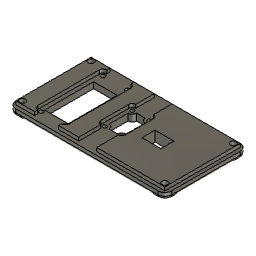
box+top (Autodesk Fusion 360 design; units mm, degrees)
Autodesk Fusion 360 part; units mm, degrees
note: some values were not read from the file. Set by a fixed rule: which face or edge a step refers to.
sketch "box dimensions" plane through (0, 0, 0) normal (0, 0, 1) x (1, 0, 0)
  line L0 (104.14, -1.27) -> (-6.35, -1.27)
  line L1 (-6.35, -1.27) -> (-6.35, 54.61)
  line L2 (-6.35, 54.61) -> (104.14, 54.61)
  line L3 (104.14, 54.61) -> (104.14, -1.27)
  line L4 (101.6, 57.15) -> (-3.81, 57.15)
  line L5 (-8.89, 52.07) -> (-8.89, 1.27)
  line L6 (-3.81, -3.81) -> (101.6, -3.81)
  arc A0 (106.68, 52.07) -> (101.6, 57.15) centre (101.6, 52.07) ccw
  line L7 (106.68, 1.27) -> (106.68, 52.07)
  arc A1 (-3.81, 57.15) -> (-8.89, 52.07) centre (-3.81, 52.07) ccw
  arc A2 (101.6, -3.81) -> (106.68, 1.27) centre (101.6, 1.27) ccw
  arc A3 (-8.89, 1.27) -> (-3.81, -3.81) centre (-3.81, 1.27) ccw
  circle A4 centre (-3.81, 52.07) radius 2.159
  circle A5 centre (-3.81, 1.27) radius 2.159
  circle A6 centre (101.6, 1.27) radius 2.159
  circle A7 centre (-3.81, 52.07) radius 2.159
  circle A8 centre (-3.81, 1.27) radius 2.159
  circle A9 centre (101.6, 52.07) radius 2.159
  line L8 (68.834, 6.35) -> (68.834, 4.9748)
  line L9 (-0.254, 53.594) -> (64.6598, 53.594)
  line L10 (71.12, 6.35) -> (68.834, 6.35)
  line L11 (-2.159, 2.921) -> (-2.159, 12.319)
  line L12 (104.14, 54.61) -> (-6.35, 54.61)
  line L13 (-2.159, 12.319) -> (-0.254, 12.319)
  line L14 (104.14, -1.27) -> (104.14, 54.61)
  line L15 (-0.254, -0.254) -> (-0.254, 2.921)
  line L16 (98.044, 0) -> (71.12, 0)
  line L17 (71.12, 53.34) -> (98.044, 53.34)
  line L18 (-6.35, 44.069) -> (-0.254, 44.069)
  line L19 (98.044, 53.34) -> (98.044, 0)
  line L20 (-6.35, -1.27) -> (104.14, -1.27)
  line L21 (-0.254, 30.861) -> (-6.35, 30.861)
  line L22 (66.294, -0.254) -> (-0.254, -0.254)
  line L23 (-0.254, 2.921) -> (-2.159, 2.921)
  line L24 (-0.254, 44.069) -> (-0.254, 53.594)
  line L25 (71.12, 0) -> (71.12, 6.35)
  line L26 (66.294, 2.4348) -> (66.294, -0.254)
  line L27 (71.12, 50.8704) -> (71.12, 53.34)
  line L28 (-0.254, 12.319) -> (-0.254, 30.861)
  line L29 (-6.35, 30.861) -> (-6.35, -1.27)
  line L30 (66.294, 50.8704) -> (71.12, 50.8704)
  line L31 (-6.35, 54.61) -> (-6.35, 44.069)
  line L32 (64.6598, 53.594) -> (66.294, 50.8704)
  line L33 (68.834, 4.9748) -> (66.294, 2.4348)
  circle A10 centre (101.6, 52.07) radius 2.159
  circle A11 centre (101.6, 1.27) radius 2.159
extrude "Extrude1" add sketch "box dimensions" along normal blind 2.54 contours L0 L1 L2 L3 L8 L9 L10 L11 L12 L13 L14 L15 L16 L17 L18 L19 L20 L21 L22 L23 L24 L25 L26 L27 L28 L29 L30 L31 L32 L33 | L1 L8 L9 L10 L11 L13 L15 L16 L17 L18 L19 L21 L22 L23 L24 L25 L26 L27 L28 L30 L32 L33 | L4 L5 L6 A0 L7 A1 A2 A3
extrude "Extrude2" add sketch "box dimensions" along normal blind 5.08 contours L0 L1 L2 L3 L8 L9 L10 L11 L12 L13 L14 L15 L16 L17 L18 L19 L20 L21 L22 L23 L24 L25 L26 L27 L28 L29 L30 L31 L32 L33 | L1 L8 L9 L10 L11 L13 L15 L16 L17 L18 L19 L21 L22 L23 L24 L25 L26 L27 L28 L30 L32 L33
move_face "OffsetFaces1" offset 2.54 1 faces at (65.8149, 18.5156, 0)
hole "Hole2" at (-3.81, 1.27, 0) at (-3.81, 52.07, 0) at (101.6, 52.07, 0) at (101.6, 1.27, 0) direction (0, 0, -1) diameter 8.763 depth 2.54 tip angle 180
fillet "Fillet1" radius 2.54 8 edges at (48.895, 57.15, -2.54) (-7.4021, 55.6621, -2.54) (-8.89, 26.67, -2.54) (-7.4021, -2.3221, -2.54) (48.895, -3.81, -2.54) (105.1921, -2.3221, -2.54) (106.68, 26.67, -2.54) (105.1921, 55.6621, -2.54) 1 faces at (32.5915, 34.4064, -2.54)
sketch "featherwing exact dimensions" plane through (0, 0, 5.08) normal (0, 0, 1) x (1, 0, 0)
  line L0 (25.4, 52.07) -> (7.62, 52.07)
  arc A0 (27.94, 49.53) -> (25.4, 52.07) centre (25.4, 49.53) ccw
  line L1 (27.94, 3.81) -> (27.94, 49.53)
  arc A1 (25.4, 1.27) -> (27.94, 3.81) centre (25.4, 3.81) ccw
  arc A2 (5.08, 3.81) -> (7.62, 1.27) centre (7.62, 3.81) ccw
  line L2 (5.08, 49.53) -> (5.08, 3.81)
  arc A3 (7.62, 52.07) -> (5.08, 49.53) centre (7.62, 49.53) ccw
  line L3 (7.62, 1.27) -> (25.4, 1.27)
  line L4 (25.019, 42.0878) -> (8.001, 42.0878)
  line L5 (25.019, 6.2992) -> (25.019, 42.0878)
  line L6 (8.001, 6.2992) -> (25.019, 6.2992)
  line L7 (8.001, 42.0878) -> (8.001, 6.2992)
  circle A4 centre (7.62, 49.53) radius 1.27
  circle A5 centre (25.4, 49.53) radius 1.27
  circle A6 centre (25.4, 3.81) radius 1.27
  circle A7 centre (7.62, 3.81) radius 1.27
  circle A8 centre (101.6, 1.27) radius 2.159
  circle A9 centre (101.6, 52.07) radius 2.159
  circle A10 centre (-3.81, 1.27) radius 2.159
  circle A11 centre (-3.81, 52.07) radius 2.159
  line L8 (-6.35, 54.61) -> (-6.35, -1.27)
  line L9 (-6.35, -1.27) -> (104.14, -1.27)
  line L10 (104.14, -1.27) -> (104.14, 54.61)
  line L11 (104.14, 54.61) -> (-6.35, 54.61)
  circle A12 centre (7.62, 49.53) radius 1.905
  circle A13 centre (25.4, 49.53) radius 1.905
  circle A14 centre (25.4, 3.81) radius 1.905
  circle A15 centre (7.62, 3.81) radius 1.905
  dimension "d75" = 3.81
  dimension "d76" = 3.81
  dimension "d77" = 3.81
  dimension "d78" = 3.81
  constraint concentric A3 A12
  constraint concentric A0 A13
  constraint concentric A6 A14
  constraint concentric A2 A15
  measures "d75" diameter of A12
  measures "d76" diameter of A13
  measures "d77" diameter of A14
  measures "d78" diameter of A15
extrude "Extrude3" cut sketch "featherwing exact dimensions" against normal blind 12.7 contours A4 | A5 | A6 | A7
extrude "Extrude4" cut sketch "featherwing exact dimensions" against normal blind 10.16 contours L4 L5 L6 L7
move_face "OffsetFaces2" offset -0.254 4 faces at (25.019, 18.2287, 2.54) (19.3463, 6.2992, 0) (8.001, 30.1583, 2.54) (13.6737, 42.0878, 0)
extrude "Extrude5" cut sketch "featherwing exact dimensions" against normal blind 5.08 contours L0 A0 L1 A1 A2 L2 A3 L3 | A12 | A13 | A14 | A15
move_face "OffsetFaces3" offset -0.254 4 faces at (27.94, 19.05, 3.3867) (13.5467, 52.07, 1.6933) (13.5467, 1.27, 3.3867) (5.08, 34.29, 3.3867)
move_face "OffsetFaces4" offset -0.254 4 faces at (26.6637, 3.6835, -0.8467) (26.6637, 49.4035, -0.8467) (8.8884, 49.5933, -0.8467) (8.8837, 3.6835, -0.8467)
sketch "aht20 exact dimensions" plane through (0, 0, 5.08) normal (0, 0, 1) x (1, 0, 0)
  line L0 (53.34, 40.64) -> (40.64, 40.64)
  line L1 (38.1, 38.1) -> (38.1, 17.78)
  line L2 (55.88, 17.78) -> (55.88, 38.1)
  arc A0 (38.1, 17.78) -> (40.64, 15.24) centre (40.64, 17.78) ccw
  arc A1 (55.88, 38.1) -> (53.34, 40.64) centre (53.34, 38.1) ccw
  arc A2 (53.34, 15.24) -> (55.88, 17.78) centre (53.34, 17.78) ccw
  arc A3 (40.64, 40.64) -> (38.1, 38.1) centre (40.64, 38.1) ccw
  line L3 (40.64, 15.24) -> (53.34, 15.24)
  circle A4 centre (40.64, 17.78) radius 1.27
  circle A5 centre (40.64, 38.1) radius 1.27
  circle A6 centre (53.34, 38.1) radius 1.27
  circle A7 centre (53.34, 17.78) radius 1.27
extrude "Extrude6" cut sketch "aht20 exact dimensions" against normal blind 2.54
extrude "Extrude7" cut 4 faces at (40.4853, 18.1741, 5.08) (40.8517, 37.7334, 5.08) (53.1853, 38.4392, 5.08) (53.1853, 18.1741, 5.08) along direction (0, 0, -1) blind 7.62
move_face "OffsetFaces5" offset -0.254 4 faces at (38.1, 31.3267, 4.2333) (44.8733, 15.24, 4.2333) (55.88, 24.5533, 3.3867) (49.1067, 40.64, 4.2333)
move_face "OffsetFaces6" offset -0.127 4 faces at (52.2563, 37.4378, -0.8467) (40.8605, 39.3507, 0.8467) (52.2563, 17.1178, -0.8467) (39.5563, 17.1178, -0.8467)
sketch "Sketch4" plane through (0, 0, 0) normal (0, 0, 1) x (-1, 0, 0)
  arc A0 (-4.826, -3.556) -> (-7.366, -1.016) centre (-7.366, -3.556) ccw
  line L0 (-7.366, -1.016) -> (-25.654, -1.016)
  arc A1 (-25.654, -1.016) -> (-28.194, -3.556) centre (-25.654, -3.556) ccw
  line L1 (-28.194, -3.556) -> (-28.194, -49.784)
  arc A2 (-28.194, -49.784) -> (-25.654, -52.324) centre (-25.654, -49.784) ccw
  line L2 (-25.654, -52.324) -> (-7.366, -52.324)
  arc A3 (-7.366, -52.324) -> (-4.826, -49.784) centre (-7.366, -49.784) ccw
  line L3 (-4.826, -49.784) -> (-4.826, -3.556)
  line L4 (-7.747, -42.3418) -> (-25.273, -42.3418)
  line L5 (-25.273, -42.3418) -> (-25.273, -6.0452)
  line L6 (-25.273, -6.0452) -> (-7.747, -6.0452)
  line L7 (-7.747, -6.0452) -> (-7.747, -42.3418)
  circle A4 centre (-7.62, -3.81) radius 1.524
  circle A5 centre (-25.4, -49.53) radius 1.524
  circle A6 centre (-7.62, -49.53) radius 1.524
  circle A7 centre (-25.4, -3.81) radius 1.524
  point P0 (-53.34, -38.1)
  point P1 (-40.64, -38.1)
  point P2 (-40.64, -17.78)
  point P3 (-53.34, -17.78)
hole "Hole3" at (53.34, 17.78, 0) at (53.34, 38.1, 0) at (40.64, 17.78, 0) at (40.64, 38.1, 0) direction (0, 0, -1) diameter 7.62 depth 2.54 tip angle 180
sketch "Sketch5" plane through (0, 0, -2.54) normal (0, 0, -1) x (1, 0, 0)
  circle A0 centre (40.64, -17.78) radius 3.81
  circle A1 centre (53.34, -17.78) radius 3.81
  circle A2 centre (53.34, -38.1) radius 3.81
  circle A3 centre (40.64, -38.1) radius 3.81
  line L0 (7.747, -6.0452) -> (25.273, -6.0452)
  line L1 (25.273, -6.0452) -> (25.273, -42.3418)
  line L2 (25.273, -42.3418) -> (7.747, -42.3418)
  line L3 (7.747, -42.3418) -> (7.747, -6.0452)
  circle A4 centre (25.4, -3.81) radius 1.524
  circle A5 centre (25.4, -49.53) radius 1.524
  circle A6 centre (7.62, -3.81) radius 1.524
  circle A7 centre (7.62, -49.53) radius 1.524
  arc A8 (95.1614, 1.27) -> (104.14, -7.7086) centre (101.6, -1.27) ccw
  line L4 (95.1614, 1.27) -> (2.6286, 1.27)
  arc A9 (-6.35, -7.7086) -> (2.6286, 1.27) centre (-3.81, -1.27) ccw
  line L5 (-6.35, -7.7086) -> (-6.35, -45.6314)
  arc A10 (2.6286, -54.61) -> (-6.35, -45.6314) centre (-3.81, -52.07) ccw
  line L6 (2.6286, -54.61) -> (95.1614, -54.61)
  arc A11 (104.14, -45.6314) -> (95.1614, -54.61) centre (101.6, -52.07) ccw
  line L7 (104.14, -45.6314) -> (104.14, -7.7086)
  line L8 (40.64, -17.78) -> (53.34, -17.78)
  line L9 (53.34, -17.78) -> (53.34, -38.1)
  line L10 (53.34, -38.1) -> (40.64, -38.1)
  line L11 (40.64, -38.1) -> (40.64, -17.78)
  line L12 (49.53, -21.59) -> (49.53, -34.29)
  line L13 (49.53, -34.29) -> (44.45, -34.29)
  line L14 (44.45, -34.29) -> (44.45, -21.59)
  line L15 (44.45, -21.59) -> (49.53, -21.59)
  dimension "d32" = 3.81
  constraint horizontal L8
  constraint vertical L9
  constraint horizontal L10
  constraint vertical L11
  constraint coincident A2.centre L9.end
  constraint coincident A0.centre L8.start
extrude "Extrude8" cut sketch "Sketch5" against normal blind 17.78 contours L12 L13 L14 L15
fillet "Fillet2" radius 1.27 4 edges at (49.7878, 16.4022, -2.54) (37.0878, 16.4022, -2.54) (37.0878, 36.7222, -2.54) (49.7878, 36.7222, -2.54)
fillet "Fillet3" radius 0.635 4 edges at (7.747, 24.1935, -2.54) (16.51, 6.0452, -2.54) (25.273, 24.1935, -2.54) (16.51, 42.3418, -2.54)
fillet "Fillet4" radius 0.635 4 edges at (44.45, 27.94, -2.54) (46.99, 34.29, -2.54) (46.99, 21.59, -2.54) (49.53, 27.94, -2.54)
sketch "Sketch6" plane through (0, 0, -2.54) normal (0, 0, -1) x (1, 0, 0)
  line L0 (50.165, -21.7456) -> (50.165, -34.1344)
  arc A0 (49.3744, -34.925) -> (50.165, -34.1344) centre (53.34, -38.1) ccw
  line L1 (49.3744, -34.925) -> (44.6056, -34.925)
  arc A1 (43.815, -34.1344) -> (44.6056, -34.925) centre (40.64, -38.1) ccw
  line L2 (43.815, -34.1344) -> (43.815, -21.7456)
  arc A2 (44.6056, -20.955) -> (43.815, -21.7456) centre (40.64, -17.78) ccw
  line L3 (44.6056, -20.955) -> (49.3744, -20.955)
  arc A3 (50.165, -21.7456) -> (49.3744, -20.955) centre (53.34, -17.78) ccw
  arc A4 (95.1614, 1.27) -> (104.14, -7.7086) centre (101.6, -1.27) ccw
  line L4 (95.1614, 1.27) -> (2.6286, 1.27)
  arc A5 (-6.35, -7.7086) -> (2.6286, 1.27) centre (-3.81, -1.27) ccw
  line L5 (-6.35, -7.7086) -> (-6.35, -45.6314)
  arc A6 (2.6286, -54.61) -> (-6.35, -45.6314) centre (-3.81, -52.07) ccw
  line L6 (2.6286, -54.61) -> (95.1614, -54.61)
  arc A7 (104.14, -45.6314) -> (95.1614, -54.61) centre (101.6, -52.07) ccw
  line L7 (104.14, -45.6314) -> (104.14, -7.7086)
  circle A8 centre (7.62, -49.53) radius 1.524
  circle A9 centre (7.62, -3.81) radius 1.524
  circle A10 centre (25.4, -49.53) radius 1.524
  circle A11 centre (25.4, -3.81) radius 1.524
  line L8 (25.908, -42.9768) -> (7.112, -42.9768)
  line L9 (7.112, -42.9768) -> (7.112, -5.4102)
  line L10 (7.112, -5.4102) -> (25.908, -5.4102)
  line L11 (25.908, -5.4102) -> (25.908, -42.9768)
  line L12 (64.135, -16.764) -> (78.105, -16.764)
  line L13 (78.105, -16.764) -> (78.105, -36.576)
  line L14 (78.105, -36.576) -> (64.135, -36.576)
  line L15 (64.135, -36.576) -> (64.135, -16.764)
  line L16 (64.135, -16.764) -> (78.105, -36.576)
  line L17 (78.105, -16.764) -> (64.135, -36.576)
  line L18 (104.14, -26.67) -> (-6.35, -26.67)
  point P0 (104.14, -26.67)
  dimension "d41" = 13.97
  dimension "d42" = 19.812
  constraint horizontal L12
  constraint vertical L13
  constraint horizontal L14
  constraint vertical L15
  constraint midpoint L7 P0
  constraint coincident P0 L18.start
  constraint midpoint L5 L18.end
  measures "d41" distance of L12.start L12.end
  measures "d42" distance of L12.start L14.end
extrude "Extrude9" cut sketch "Sketch6" against normal blind 15.24 contours L15 L17 L18 | L15 L16 L18 | L14 L16 L17 | L12 L16 L17 | L13 L16 L18 | L13 L17 L18
extrude "Extrude10" add 1 faces at (19.0536, 44.4517, 0) along direction (0, 0, 1) blind 5.08
extrude "Extrude11" add 2 faces at (13.589, 42.3418, 1.6933) (19.431, 42.3418, -1.27) along direction (0, -1, 0) blind 36.322
extrude "Extrude12" cut sketch "featherwing exact dimensions" against normal blind 2.54 contours L0 A0 L1 A1 A2 L2 A3 L3 | A12 | A13 | A14 | A15
extrude "Extrude13" cut sketch "featherwing exact dimensions" against normal blind 5.08 contours L4 L5 L6 L7
extrude "Extrude14" cut 1 faces at (13.6737, 18.2287, 0) along direction (0, 0, -1) blind 2.54
extrude "Extrude15" cut sketch "featherwing exact dimensions" against normal blind 5.08 contours L0 A0 L1 A1 A2 L2 A3 L3 | A12 | A13 | A14 | A15
move_face "OffsetFaces7" offset -0.254 8 faces at (5.08, 34.29, 3.3867) (13.5467, 52.07, 1.6933) (5.7817, 51.2828, 1.6933) (7.1393, 1.3159, 1.6933) (13.5467, 1.27, 3.3867) (26.9701, 1.8134, 1.6933) (27.94, 34.29, 1.6933) (27.9371, 49.6509, 3.3867)
move_face "OffsetFaces8" offset -0.254 4 faces at (25.019, 18.2287, -0.635) (19.3463, 42.0878, -0.635) (8.001, 30.1583, -0.635) (13.6737, 6.2992, -0.635)
extrude "Extrude16" add 1 faces at (68.7917, 16.764, 2.54) along direction (0, 1, 0) blind 3.81
extrude "Extrude17" add 1 faces at (73.4483, 36.576, 2.54) along direction (0, -1, 0) blind 3.81
extrude "Extrude18" add 1 faces at (73.4483, 32.766, 2.54) along direction (0, -1, 0) blind 1.27
extrude "Extrude19" add 1 faces at (68.7917, 20.574, 2.54) along direction (0, 1, 0) blind 1.27
delete_face "DeleteFace1" 1 faces at (49.4431, 35.2301, -2.517)
delete_face "DeleteFace2" 1 faces at (48.8038, 16.0372, -2.5207)
delete_face "DeleteFace3" 1 faces at (45.1449, 36.2779, -2.5207)
delete_face "DeleteFace4" 1 faces at (43.7807, 21.0771, -2.4257)
move_face "OffsetFaces9" offset 1.27 4 faces at (53.5299, 34.2947, -0.8467) (52.9606, 13.9889, -1.6933) (42.4621, 41.446, -1.6933) (40.8299, 13.9747, -0.8467)
fillet "Fillet5" radius 0.635 4 faces at (54.8737, 40.1247, -1.6933) (54.8737, 19.8047, -1.6933) (42.1737, 19.8047, -1.6933) (42.1737, 40.1247, -1.6933)
move_face "OffsetFaces10" offset 2.54 1 faces at (13.9664, 44.4517, 0)
extrude "Extrude20" cut 1 faces at (13.5467, 1.016, 4.2333) along direction (0, -1, 0) blind 7.62
extrude "Extrude21" cut 1 faces at (19.4733, 52.324, 3.3867) along direction (0, 1, 0) blind 7.62
extrude "Extrude22" cut sketch "featherwing exact dimensions" against normal blind 12.7 from surface at -5.08 contours A12 | A13 | A14 | A15
delete_face "DeleteFace5" 1 faces at (43.9626, 25.6809, -2.5226)
delete_face "DeleteFace6" 1 faces at (48.1517, 34.7568, -2.5173)
delete_face "DeleteFace7" 1 faces at (48.1517, 21.1232, -2.5173)
delete_face "DeleteFace8" 1 faces at (49.8475, 30.0567, -2.4549)
move_face "OffsetFaces11" offset 5.08 1 faces at (44.45, 30.0567, 0.8467)
sketch "Sketch7" plane through (0, 0, -2.54) normal (0, 0, -1) x (1, 0, 0)
  circle A0 centre (53.34, -17.78) radius 3.175
  line L0 (78.105, -21.844) -> (78.105, -31.496)
  line L1 (78.105, -31.496) -> (64.135, -31.496)
  line L2 (64.135, -31.496) -> (64.135, -21.844)
  line L3 (64.135, -21.844) -> (78.105, -21.844)
  circle A1 centre (40.64, -17.78) radius 3.175
  circle A2 centre (25.4, -49.53) radius 1.905
  circle A3 centre (7.62, -49.53) radius 1.905
  circle A4 centre (40.64, -38.1) radius 3.175
  line L4 (25.908, -5.646) -> (25.908, -42.9768)
  line L5 (25.908, -42.9768) -> (7.112, -42.9768)
  line L6 (7.112, -42.9768) -> (7.112, -5.646)
  arc A5 (8.6536, -5.4102) -> (7.112, -5.646) centre (7.62, -3.81) ccw
  line L7 (8.6536, -5.4102) -> (24.3664, -5.4102)
  arc A6 (25.908, -5.646) -> (24.3664, -5.4102) centre (25.4, -3.81) ccw
  line L8 (2.6286, -54.61) -> (95.1614, -54.61)
  arc A7 (104.14, -45.6314) -> (95.1614, -54.61) centre (101.6, -52.07) ccw
  line L9 (104.14, -45.6314) -> (104.14, -7.7086)
  arc A8 (95.1614, 1.27) -> (104.14, -7.7086) centre (101.6, -1.27) ccw
  line L10 (95.1614, 1.27) -> (2.6286, 1.27)
  arc A9 (-6.35, -7.7086) -> (2.6286, 1.27) centre (-3.81, -1.27) ccw
  line L11 (-6.35, -7.7086) -> (-6.35, -45.6314)
  arc A10 (2.6286, -54.61) -> (-6.35, -45.6314) centre (-3.81, -52.07) ccw
  circle A11 centre (53.34, -38.1) radius 3.175
  line L12 (40.64, -38.1) -> (53.34, -38.1)
  line L13 (53.34, -38.1) -> (53.34, -17.78)
  line L14 (53.34, -17.78) -> (40.64, -17.78)
  line L15 (40.64, -17.78) -> (40.64, -38.1)
  constraint horizontal L12
  constraint vertical L13
  constraint horizontal L14
  constraint vertical L15
  constraint coincident A0.centre L13.end
  constraint coincident A4.centre L12.start
extrude "Extrude23" cut sketch "Sketch7" against normal blind 7.62 contours A0 A1 A4 A11 L12 L13 L14 L15
extrude "Extrude24" cut 1 faces at (44.7887, 14.986, 4.2333) along direction (0, -1, 0) blind 25.4
extrude "Extrude25" cut 1 faces at (49.1913, 40.894, 4.2333) along direction (0, 1, 0) blind 20.32
